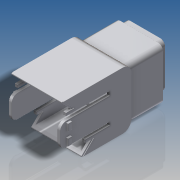
# Autodesk Inventor part: 99534-White
Saved by Autodesk Inventor 2016 SP2 (Build 200236200, 236)
## iProperties
Created: 2015-09-02
Part Number: 99534-White
Material: ABS Plastic
Document SubType Name: Modeling
Designer: D. Kohfeld
Density: 1.06 g/cm^3
Appearance: White
Mass: 4.49235 g
Surface Area: 69.1269 cm^2
Volume: 4.23807 cm^3
Author: D. Kohfeld
Autodesk Inventor part; units mm, degrees
ref_plane "YZ Plane" through (0, 0, 0) normal (1, 0, 0) x (0, 1, 0)
ref_plane "XZ Plane" through (0, 0, 0) normal (0, 1, 0) x (-1, 0, 0)
sketch "Sketch2" plane through (0, 0, 0) normal (1, 0, 0) x (0, 1, 0)
  line L0 (11.6, 28) -> (11.6, 3.6)
  arc A0 (8, 0) -> (11.6, 3.6) centre (8, 3.6) ccw
  line L1 (8, 0) -> (-8, 0)
  arc A1 (-11.6, 3.6) -> (-8, 0) centre (-8, 3.6) ccw
  line L2 (-11.6, 3.6) -> (-11.6, 20)
  line L3 (-11.2, 20) -> (-7.2, 16)
  line L4 (-6, 18.8) -> (-6, 8.8)
  line L5 (-6, 8.8) -> (-4.8, 8.8)
  line L6 (-4.8, 8.8) -> (-4.8, 26.4)
  arc A2 (-2.4, 28.8) -> (-4.8, 26.4) centre (-2.4, 26.4) ccw
  line L7 (-2.4, 28.8) -> (2, 28.8)
  arc A3 (4.4, 26.4) -> (2, 28.8) centre (2, 26.4) ccw
  line L8 (4.4, 26.4) -> (4.4, 8.8)
  line L9 (4.4, 8.8) -> (6, 8.8)
  line L10 (6, 8.8) -> (6, 26.4)
  line L11 (7.2, 24) -> (11.2, 28)
  line L12 (11.2, 28) -> (11.6, 28)
  line L13 (-11.2, 20) -> (-11.6, 20)
  line L14 (7.2, 24) -> (7.2, 26.4)
  line L15 (7.2, 26.4) -> (6, 26.4)
  line L16 (-7.2, 16) -> (-7.2, 18.8)
  line L17 (-7.2, 18.8) -> (-6, 18.8)
  line L18 (-10.4, 19.2) -> (-10.4, 2)
  line L19 (-10.4, 2) -> (10.4, 2)
  line L20 (10.4, 2) -> (10.4, 27.2)
  point P0 (0, 0)
  point P1 (0, 0)
  dimension "d0" = 5.6
  dimension "d1" = 5.6
  dimension "d2" = 1.2
  dimension "d3" = 0.4
  dimension "d4" = 45
  dimension "d5" = 28
  dimension "d6" = 20
  dimension "d7" = 8.8
  dimension "d8" = 23.2
  dimension "d9" = 1.2
  dimension "d10" = 1.6
  dimension "d11" = 3.6
  dimension "d12" = 17.6
  dimension "d13" = 10
  dimension "d14" = 28.8
  dimension "d15" = 2.4
  dimension "d16" = 1.2
  dimension "d17" = 1.2
  dimension "d18" = 2
  constraints: 42 end point, 10 vertical, 9 horizontal, 8 point on circle, 8 tangent, 4 centre point, 2 equal radius, 2 parallel, 2 point on line, 1 coincident, 1 horizontal alignment, 1 midpoint, 1 perpendicular
  measures "d0" distance between parallel lines of L0 L10
  measures "d1" distance between parallel lines of L2 L4
  measures "d2" distance between parallel lines of L16 L4
  measures "d3" distance from line of L3.start L2
  measures "d4" angle of L2 L3
  measures "d5" distance from line of L0.start L1
  measures "d6" distance from line of L2.end L1
  measures "d7" distance between parallel lines of L5 L1
  measures "d8" distance between parallel lines of L2 L0
  measures "d9" distance between parallel lines of L6 L4
  measures "d10" distance between parallel lines of L10 L8
  measures "d11" radius of A1
  measures "d12" distance of L9.end L10.end
  measures "d13" distance of L4.start L4.end
  measures "d14" distance between parallel lines of L7 L1
  measures "d15" radius of A2
  measures "d16" distance between parallel lines of L2 L18
  measures "d17" distance between parallel lines of L0 L20
  measures "d18" distance between parallel lines of L19 L1
extrude "Extrusion1" add sketch "Sketch2" along normal mid plane 20.8
extrude "Extrusion2" cut sketch "Sketch2" along normal mid plane 18.4 contours L20 L19 L18 L3 L16 L17 L4 L5 L6 A2 L7 A3 L8 L9 L10 L15 L14 L11
sketch "Sketch3" plane through (10.4, 0, 0) normal (1, 0, 0) x (0, 0, -1)
  line L0 (-28, 11.6) -> (-28, 11.2) projected
  line L1 (-28, 11.2) -> (-24, 7.2) projected
  line L2 (-28.8, 2) -> (-28.8, -2.4) projected
  line L3 (-16, -7.2) -> (-20, -11.2) projected
  line L4 (-20, -11.2) -> (-20, -11.6) projected
  line L5 (-20, -11.6) -> (-3.6, -11.6) projected
  line L6 (-3.6, 11.6) -> (-28, 11.6) projected
  line L7 (-26.4, 3.8) -> (-24.8, 3.8)
  line L8 (-24.8, 3.8) -> (-24.8, 1)
  line L9 (-24.8, 1) -> (-26.4, 1)
  line L10 (-26.4, 1) -> (-26.4, 3.8)
  line L11 (-26.4, -1.4) -> (-24.8, -1.4)
  line L12 (-24.8, -1.4) -> (-24.8, -4.2)
  line L13 (-24.8, -4.2) -> (-26.4, -4.2)
  line L14 (-26.4, -4.2) -> (-26.4, -1.4)
  line L15 (-27.6, 11.6) -> (-23.2, 7.2)
  line L16 (-23.2, 7.2) -> (-24, 7.2)
  line L17 (-19.6, -11.6) -> (-15.2, -7.2)
  line L18 (-15.2, -7.2) -> (-16, -7.2)
  line L19 (-26.4, -1.4) -> (-24.8, 1) construction
  point P0 (0, 0)
  point P1 (-28.8, -0.2)
  point P2 (-25.6, -0.2)
  dimension "d23" = 0.8
  dimension "d24" = 2.8
  dimension "d25" = 1.6
  dimension "d26" = 2.4
  dimension "d27" = 2.4
  constraints: 26 end point, 5 parallel, 4 horizontal, 3 equal length, 3 perpendicular, 2 midpoint, 2 point on line, 1 horizontal alignment, 1 vertical alignment
  measures "d23" distance of L15.end L1.end
  measures "d24" distance of L7.end L8.end
  measures "d25" distance of L7.start L7.end
  measures "d26" distance between parallel lines of L11 L9
  measures "d27" distance between parallel lines of L14 L2
extrude "Extrusion3" cut sketch "Sketch3" against normal blind 0.2 contours L6 L15 L16 L1 L0 | L18 L17 L5 L4 L3
extrude "Extrusion4" add sketch "Sketch3" along normal blind 0.8 contours L7 L8 L9 L10 | L11 L12 L13 L14
mirror "Mirror1" about plane through (0, 0, 0) normal (1, 0, 0) of "Extrusion4", "Extrusion3"
ref_plane "Work Plane1" through (10.4, 8, -13.6) normal (0, 0, -1) x (-1, 0, 0)
sketch "Sketch4" plane through (10.4, 8, -13.6) normal (0, 0, -1) x (-1, 0, 0)
  line L0 (2.8, 2.4) -> (18, 2.4)
  line L1 (20, 0.4) -> (20, -16.4)
  line L2 (18, -18.4) -> (2.8, -18.4)
  line L3 (0.8, -16.4) -> (0.8, 0.4)
  line L4 (4.4, 2) -> (16.4, 2)
  line L5 (18.4, 0) -> (18.4, -14)
  line L6 (16.4, -16) -> (4.4, -16)
  line L7 (2.4, -14) -> (2.4, 0)
  line L8 (5.36, 0.56) -> (15.44, 0.56)
  line L9 (16.4, -0.4) -> (16.4, -14)
  line L10 (4.4, -14) -> (4.4, -0.4)
  arc A0 (2.8, 2.4) -> (0.8, 0.4) centre (2.8, 0.4) ccw
  arc A1 (20, 0.4) -> (18, 2.4) centre (18, 0.4) ccw
  arc A2 (18, -18.4) -> (20, -16.4) centre (18, -16.4) ccw
  arc A3 (0.8, -16.4) -> (2.8, -18.4) centre (2.8, -16.4) ccw
  arc A4 (4.4, 2) -> (2.4, 0) centre (4.4, 0) ccw
  arc A5 (18.4, 0) -> (16.4, 2) centre (16.4, 0) ccw
  arc A6 (2.4, -14) -> (4.4, -16) centre (4.4, -14) ccw
  arc A7 (16.4, -16) -> (18.4, -14) centre (16.4, -14) ccw
  arc A8 (5.36, 0.56) -> (4.4, -0.4) centre (5.36, -0.4) ccw
  arc A9 (16.4, -0.4) -> (15.44, 0.56) centre (15.44, -0.4) ccw
  line L11 (5.2, -14) -> (5.2, -11.6)
  line L12 (5.2, -11.6) -> (15.6, -11.6)
  line L13 (15.6, -11.6) -> (15.6, -14)
  line L14 (16.4, -14) -> (15.6, -14)
  line L15 (5.2, -14) -> (4.4, -14)
  point P0 (10.4, -8)
  point P1 (10.4, 0.56)
  point P2 (10.4, 2)
  point P3 (10.4, 2.4)
  point P4 (0.8, -8)
  dimension "d33" = 2
  dimension "d34" = 2
  dimension "d35" = 0.96
  dimension "d36" = 2.4
  dimension "d38" = 20.8
  dimension "d39" = 18
  dimension "d41" = 14.56
  dimension "d42" = 10.4
  dimension "d43" = 12
  dimension "d44" = 2
  dimension "d45" = 16
  dimension "d46" = 19.2
  dimension "d47" = 2.4
  constraints: 32 end point, 20 point on circle, 20 tangent, 10 centre point, 7 equal radius, 7 parallel, 4 horizontal, 4 midpoint, 3 perpendicular, 3 vertical alignment, 2 equal length, 2 vertical, 1 horizontal alignment
  measures "d33" radius of A0
  measures "d34" radius of A4
  measures "d35" radius of A8
  measures "d36" distance between parallel lines of L6 L2
  measures "d38" distance between parallel lines of L2 L0
  measures "d39" distance between parallel lines of L6 L4
  measures "d41" distance between parallel lines of L8 L15
  measures "d42" distance of L11.end L12.end
  measures "d43" distance between parallel lines of L9 L10
  measures "d44" distance between parallel lines of L15 L6
  measures "d45" distance between parallel lines of L5 L7
  measures "d46" distance between parallel lines of L1 L3
  measures "d47" distance between parallel lines of L12 L15
extrude "Extrusion5" add sketch "Sketch4" against normal up to next contours L0 A1 L1 A2 L2 A3 L3 A0 | L4 A5 L5 A7 L6 A6 L7 A4
extrude "Extrusion6" add sketch "Sketch4" along normal blind 2.4 contours L4 A5 L5 A7 L6 A6 L7 A4
sketch "Sketch5" plane through (-9.2, -10.4, 2) normal (0, 0, 1) x (1, 0, 0)
  line L0 (1.2, 19.6) -> (17.2, 19.6)
  line L1 (17.2, 19.6) -> (17.2, 1.2)
  line L2 (17.2, 1.2) -> (1.2, 1.2)
  line L3 (1.2, 1.2) -> (1.2, 19.6)
  line L4 (2, 19.6) -> (2, 3.6)
  line L5 (2, 3.6) -> (16.4, 3.6)
  line L6 (16.4, 3.6) -> (16.4, 19.6)
  point P0 (9.2, 10.4)
  point P1 (9.2, 19.6)
  point P2 (1.2, 10.4)
  point P3 (9.2, 3.6)
  dimension "d52" = 18.4
  dimension "d53" = 16
  dimension "d54" = 14.4
  dimension "d55" = 16
  constraints: 14 end point, 3 midpoint, 2 horizontal, 2 parallel, 2 point on line, 2 vertical, 2 vertical alignment, 1 horizontal alignment, 1 perpendicular
  measures "d52" distance of L2.end L0.start
  measures "d53" distance of L0.start L0.end
  measures "d54" distance of L4.end L5.end
  measures "d55" distance of L4.start L4.end
extrude "Extrusion7" cut sketch "Sketch5" against normal blind 14
extrude "Extrusion8" cut sketch "Sketch5" against normal blind 15.6 contours L0 L6 L5 L4
fillet "Fillet1" radius 0.1 177 edges at (0, 11.6, 28) (0, 11.2, 28) (10.4, 10.5456, 1.0544) (10.4, 0, 0) (10.4, -10.5456, 1.0544) (10.4, -11.6, 11.6) (10.4, 11.6, 15.6) (10.2, 11.6, 27.8) (10.2, 11.4, 28) (10.4, 9.4, 25.4) (10.3, 11.6, 27.6) (10.2, 9.2, 26) (9.2, 7.2, 25.2) (9.8, 7.2, 26.4) (9.2, 6.6, 26.4) (9.8, 6, 26.4) (9.2, 6, 17.6) (10.4, 6.6, 26.4) (10.4, 6, 17.6) (10.4, 5.2, 8.8) (9.2, 5.2, 8.8) (10.4, 3.6971, 28.0971) (10.4, -0.2, 28.8) (10.4, -4.0971, 28.0971) (10.4, -4.8, 17.6) (10.4, 4.4, 17.6) (9.2, 3.6971, 28.0971) (9.2, -0.2, 28.8) (9.2, -4.0971, 28.0971) (9.2, -4.8, 17.6) (9.2, 4.4, 17.6) (10.8, 3.8, 26.4) (11.2, 2.4, 26.4) (10.8, 1, 26.4) (11.2, 1, 25.6) (10.8, 1, 24.8) (11.2, 2.4, 24.8) (10.8, 3.8, 24.8) (11.2, 3.8, 25.6) (10.8, -1.4, 24.8) (11.2, -1.4, 25.6) (10.8, -1.4, 26.4) (11.2, -2.8, 26.4) (10.8, -4.2, 26.4) (11.2, -4.2, 25.6) (11.2, -2.8, 24.8) (10.8, -4.2, 24.8) (9.2, -6.6, 18.8) (9.8, -6, 18.8) (9.2, -6, 13.8) (9.2, -5.4, 8.8) (10.4, -5.4, 8.8) (10.4, -6, 13.8) (10.4, -6.6, 18.8) (9.8, -7.2, 18.8) (9.2, -7.2, 17.4) (10.4, -7.2, 17) (10.2, -9.2, 18) (9.2, -8.8, 17.6) (10.4, -9.4, 17.4) (10.3, -11.6, 19.6) (10.2, -11.6, 19.8) (10.2, -11.4, 20) (0, -11.6, 20) (0, -11.2, 20) (0, -10.4, 19.2) (-10.2, -11.4, 20) (-10.2, -11.6, 19.8) (-10.2, -9.2, 18) (-9.2, -8.8, 17.6) (-9.2, -7.2, 17.4) (-9.8, -7.2, 18.8) (-9.2, -6.6, 18.8) (-10.4, -6.6, 18.8) (-9.8, -6, 18.8) (-9.2, -6, 13.8) (-9.2, -4.0971, 28.0971) (-9.2, -0.2, 28.8) (-9.2, 3.6971, 28.0971) (-9.2, 4.4, 17.6) (-9.2, -4.8, 17.6) (-10.4, -6, 13.8) (-9.2, -5.4, 8.8) (-10.4, -5.4, 8.8) (-10.4, -4.0971, 28.0971) (-10.4, -0.2, 28.8) (-10.4, 3.6971, 28.0971) (-10.4, 4.4, 17.6) (-10.4, -4.8, 17.6) (-10.4, 10.5456, 1.0544) (-10.4, 0, 0) (-10.4, -10.5456, 1.0544) (-10.4, -11.6, 11.6) (-10.4, 11.6, 15.6) (0, 10.4, 27.2) (9.2, 8.8, 25.6) (-9.2, 8.8, 25.6) (-10.2, 9.2, 26) (-10.2, 11.4, 28) (-10.3, 11.6, 27.6) (-10.2, 11.6, 27.8) (-10.4, 9.4, 25.4) (-10.4, 7.2, 24.8) (-9.2, 7.2, 25.2) (-9.8, 7.2, 26.4) (-10.4, 6.6, 26.4) (-9.8, 6, 26.4) (-9.2, 6.6, 26.4) (-9.2, 6, 17.6) (-10.4, 6, 17.6) (-9.2, 5.2, 8.8) (-10.4, 5.2, 8.8) (-10.4, -7.2, 17) (-10.3, -11.6, 19.6) (-10.4, -9.4, 17.4) (0, -9.2, 2) (-8, 0, 2) (0, -6.8, -12) (-7.2, 1.2, -12) (-5.6, -6, -13.6) (-5.2, -4.8, -13.6) (0, -3.6, -13.6) (-5.7188, 8.2788, -13.6) (0, 8.56, -13.6) (5.7188, 8.2788, -13.6) (6, 0.8, -13.6) (-6, 0.8, -13.6) (0, -3.6, -16) (-5.2, -3.6, -14.8) (-5.7188, 8.2788, -16) (0, 8.56, -16) (5.7188, 8.2788, -16) (6, 0.8, -16) (-6, 0.8, -16) (10.4, 7.2, 24.8) (-11.2, 2.4, 26.4) (-10.8, 3.8, 26.4) (-10.8, 3.8, 24.8) (-11.2, 3.8, 25.6) (-11.2, 2.4, 24.8) (-11.2, 1, 25.6) (-10.8, 1, 24.8) (-10.8, 1, 26.4) (-11.2, -2.8, 26.4) (-10.8, -1.4, 26.4) (-11.2, -1.4, 25.6) (-10.8, -1.4, 24.8) (-11.2, -2.8, 24.8) (-10.8, -4.2, 24.8) (-11.2, -4.2, 25.6) (-10.8, -4.2, 26.4) (7.2, 1.2, -12) (5.6, -6, -13.6) (5.2, -4.8, -13.6) (8, 0, 2) (0, 9.2, 2) (9.0142, -9.8142, -13.6) (0, -10.4, -13.6) (-9.0142, -9.8142, -13.6) (-9.6, 0, -13.6) (-9.0142, 9.8142, -13.6) (0, 10.4, -13.6) (9.0142, 9.8142, -13.6) (9.6, 0, -13.6) (7.4142, 9.4142, -16) (8, 1, -16) (7.4142, -7.4142, -16) (0, -8, -16) (-7.4142, -7.4142, -16) (-8, 1, -16) (-7.4142, 9.4142, -16) (0, 10, -16) (-5.2, -4.8, -16) (-5.6, -6, -16) (5.2, -4.8, -16) (5.2, -3.6, -14.8) (5.6, -6, -16)
equation "\"d25\" = wall"
equation "\"d45\" = 2 * lu"
equation "\"d53\" = 2 * lu"
equation "\"d55\" = 2 * lu"
equation "\"d60\" = lf"
equation "\"wall\" = 1.6"
equation "\"lu\" = 8"
equation "\"lf\" = 0.1"
body "Solid1"
